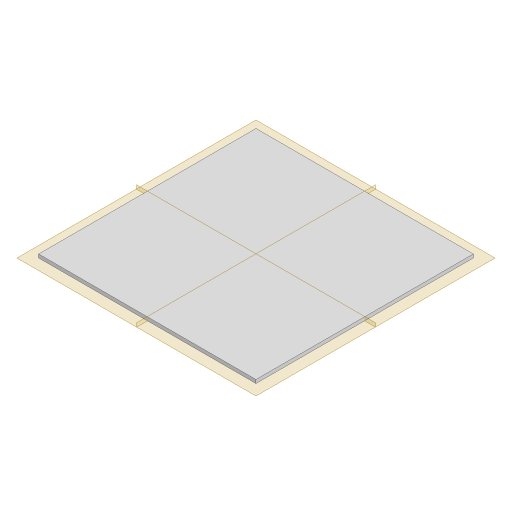
# Autodesk Inventor part: Платформа подъёмника
Saved by Autodesk Inventor 2023.2 (Build 272271030, 271C)
## iProperties
Created: 2025-03-18
Part Number: Платформа подъёмника
Material: Типовые
Document SubType Name: Modeling
Designer: Коноваленко
Density: 1 g/cm^3
Appearance: По умолчанию
Author: Коноваленко
Autodesk Inventor part; units mm, degrees
sketch "Эскиз1" plane through (0, 0, 0) normal (0, 1, 0) x (-1, 0, 0)
  line L0 (125, 125) -> (-125, 125)
  line L1 (-125, 125) -> (-125, -125)
  line L2 (-125, -125) -> (125, -125)
  line L3 (125, -125) -> (125, 125)
  line L4 (125, 125) -> (-125, -125) construction
  line L5 (-125, 125) -> (125, -125) construction
  point P0 (0, 0)
  dimension "d0" = 250
  dimension "d1" = 250
  constraints: 12 end point, 2 midpoint, 2 parallel, 1 horizontal, 1 perpendicular
  measures "d0" distance of L1.end L2.end
  measures "d1" distance of L0.end L1.end
extrude "Выдавливание1" add sketch "Эскиз1" along normal blind 4
